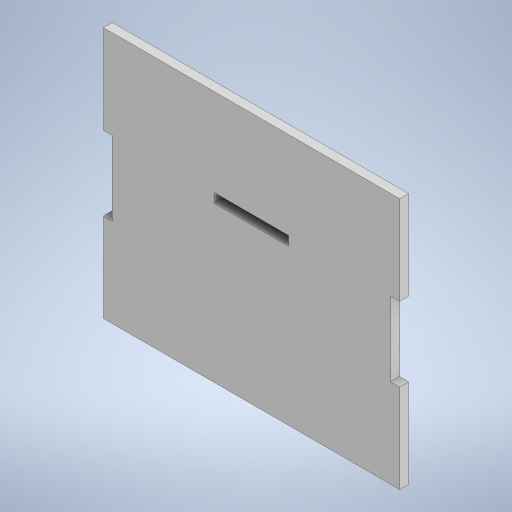
# Autodesk Inventor part: Samping
Saved by Autodesk Inventor 2023 (Build 270158000, 158)
## iProperties
Created: 2023-02-07
Part Number: Samping
Material: Generic
Document SubType Name: Modeling
Designer: Asus
Density: 1 g/cm^3
Appearance: Default
Author: Asus
Autodesk Inventor part; units mm, degrees
ref_plane "YZ Plane" through (0, 0, 0) normal (1, 0, 0) x (0, 1, 0)
ref_plane "XZ Plane" through (0, 0, 0) normal (0, 1, 0) x (-1, 0, 0)
ref_plane "XY Plane" through (0, 0, 0) normal (0, 0, 1) x (1, 0, 0)
sketch "Sketch1" plane through (0, 0, 0) normal (0, 0, 1) x (1, 0, 0)
  line L0 (0, 0) -> (100, 0)
  line L1 (100, 0) -> (100, 30)
  line L2 (100, 30) -> (97, 30)
  line L3 (97, 30) -> (97, 55)
  line L4 (97, 55) -> (100, 55)
  line L5 (100, 55) -> (100, 85)
  line L6 (100, 85) -> (0, 85)
  line L7 (0, 85) -> (0, 55)
  line L8 (0, 55) -> (3, 55)
  line L9 (3, 55) -> (3, 30)
  line L10 (3, 30) -> (0, 30)
  line L11 (0, 30) -> (0, 0)
  line L12 (50, 0) -> (50, 52.5) construction
  line L13 (50, 52.5) -> (50, 80) construction
  circle A0 centre (50, 80) radius 27.5 construction
  line L14 (50, 80) -> (50, 85) construction
  line L15 (50, 107.5) -> (50, 85) construction
  line L16 (50, 52.5) -> (50, 60.5) construction
  line L17 (50, 60.5) -> (50, 70.5) construction
  line L18 (50, 52.5) -> (50, 55.5) construction
  line L19 (50, 55.5) -> (50, 52.5) construction
  line L20 (50, 55.5) -> (62.5, 55.5)
  line L21 (62.5, 55.5) -> (62.5, 52.5)
  line L22 (62.5, 52.5) -> (37.5, 52.5)
  line L23 (37.5, 52.5) -> (37.5, 55.5)
  line L24 (37.5, 55.5) -> (50, 55.5)
  dimension "d15" = 55
  dimension "d0" = 100
  dimension "d1" = 30
  dimension "d3" = 25
  dimension "d4" = 3
  dimension "d5" = 30
  dimension "d6" = 100
  dimension "d7" = 30
  dimension "d8" = 3
  dimension "d9" = 25
  dimension "d10" = 3
  dimension "d13" = 52.5
  dimension "d14" = 27.5
  dimension "d17" = 8
  dimension "d18" = 10
  dimension "d21" = 3
  dimension "d22" = 12.5
  dimension "d23" = 3
  dimension "d24" = 25
  dimension "d25" = 3
  dimension "d26" = 52.5
  constraints: 50 end point, 13 point on line, 7 perpendicular, 3 midpoint, 2 horizontal, 1 coincident, 1 parallel, 1 vertical, 1 vertical alignment, 2 other
  measures "d0" distance of L0.start L0.end
  measures "d1" distance of L0.end L1.end
  measures "d3" distance of L2.end L3.end
  measures "d4" distance of L3.end L4.end
  measures "d5" distance of L4.end L5.end
  measures "d6" distance of L5.end L6.end
  measures "d7" distance of L6.end L7.end
  measures "d8" distance of L7.end L8.end
  measures "d9" distance of L8.end L9.end
  measures "d10" distance of L9.end L10.end
  measures "d13" distance of L12.start L12.end
  measures "d14" distance of L12.end L13.end
  measures "d17" distance of L12.end L16.end
  measures "d18" distance of L16.end L17.end
  measures "d21" distance of L18.end L19.end
  measures "d22" distance of L18.end L20.end
  measures "d23" distance of L20.end L21.end
  measures "d24" distance of L21.end L22.end
  measures "d25" distance of L22.end L23.end
  measures "d26" distance of point (50, 52.5) L12.start
extrude "Extrusion1" add sketch "Sketch1" along normal blind 3
